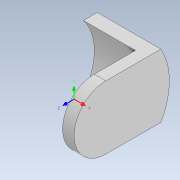
# Autodesk Inventor part: shank_board
Saved by Autodesk Inventor 2020 (Build 240168000, 168)
## iProperties
Created: 2021-01-12
Part Number: shank_board
Material: Generic
Document SubType Name: Modeling
Designer: DELL
Density: 1 g/cm^3
Appearance: Default
Author: DELL
Autodesk Inventor part; units mm, degrees
ref_plane "XZ Plane" through (0, 0, 0) normal (0, 1, 0) x (-1, 0, 0)
ref_plane "XY Plane" through (0, 0, 0) normal (0, 0, 1) x (1, 0, 0)
ref_plane "Work Plane2" through (17.5, 0, 0) normal (1, 0, 0) x (0, 1, 0)
sketch "Sketch1" plane through (0, 0, 0) normal (1, 0, 0) x (0, 1, 0)
  circle A0 centre (0, 0) radius 27.5
  line L0 (-27.5, 0) -> (-27.5, -47.6314)
  line L1 (27.5, 0) -> (27.5, -47.6314)
  arc A1 (-27.5, -35.6195) -> (27.5, -35.6195) centre (0, 0) ccw
  arc A2 (-27.5, -47.6314) -> (27.5, -47.6314) centre (0, 0) ccw
  dimension "d0" = 55
  dimension "d10" = 90
  dimension "d11" = 110
  constraints: 6 point on circle, 4 end point, 3 centre point, 3 coincident, 2 point on line, 2 tangent, 2 vertical
  measures "d0" diameter of A0
  measures "d10" diameter of A1
  measures "d11" diameter of A2
extrude "Extrusion1" add sketch "Sketch1" along normal blind 10 from surface at 17.5
extrude "Extrusion2" add sketch "Sketch1" against normal blind 45 from surface at 17.5 contours L1 A2 L0 A1
body "Solid1"
